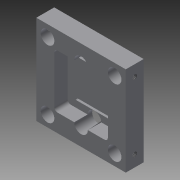
# Autodesk Inventor part: HolderEnd
Saved by Autodesk Inventor 2015 SP1 (Build 190203100, 203)
## iProperties
Created: 2014-07-11
Part Number: HolderEnd
Material: Generic
Document SubType Name: Modeling
Designer: jad211
Density: 1 g/cm^3
Appearance: Default
Author: jad211
Autodesk Inventor part; units mm, degrees
ref_plane "YZ Plane" through (0, 0, 0) normal (1, 0, 0) x (0, 1, 0)
ref_plane "XZ Plane" through (0, 0, 0) normal (0, 1, 0) x (-1, 0, 0)
ref_plane "XY Plane" through (0, 0, 0) normal (0, 0, 1) x (1, 0, 0)
sketch "Sketch1" plane through (0, 0, 0) normal (0, 1, 0) x (-1, 0, 0)
  line L0 (20, 20) -> (20, -20)
  line L1 (20, -20) -> (-20, -20)
  line L2 (-20, -20) -> (-20, 20)
  line L3 (-20, 20) -> (20, 20)
  line L4 (-15, 15) -> (-15, -15) construction
  line L5 (-15, -15) -> (15, -15) construction
  line L6 (15, -15) -> (15, 15) construction
  line L7 (15, 15) -> (-15, 15) construction
  circle A0 centre (15, 15) radius 3.05
  circle A1 centre (15, -15) radius 3.05
  circle A2 centre (-15, -15) radius 3.05
  circle A3 centre (-15, 15) radius 3.05
  line L8 (0, 0) -> (-18.5703, 0) construction
  line L9 (0, 0) -> (0, 18.05) construction
  line L10 (0, 0) -> (-18.05, 0) construction
  line L11 (8, 9) -> (-8, 9)
  line L12 (-8.5, 8.5) -> (-8.5, 8.5)
  line L13 (-8, 8) -> (8, 8)
  line L14 (8.5, 8.5) -> (8.5, 8.5)
  line L15 (8.5, 9) -> (-8.5, 8) construction
  line L16 (-8.5, 9) -> (8.5, 8) construction
  arc A4 (8.5, 8.5) -> (8, 9) centre (8, 8.5) ccw
  arc A5 (8, 8) -> (8.5, 8.5) centre (8, 8.5) ccw
  arc A6 (-8.5, 8.5) -> (-8, 8) centre (-8, 8.5) ccw
  arc A7 (-8, 9) -> (-8.5, 8.5) centre (-8, 8.5) ccw
  line L17 (8, -8) -> (-8, -8)
  line L18 (-8, -9) -> (8, -9)
  line L19 (8.5, -8) -> (-8.5, -9) construction
  line L20 (-8.5, -8) -> (8.5, -9) construction
  arc A8 (8.5, -8.5) -> (8, -8) centre (8, -8.5) ccw
  arc A9 (8, -9) -> (8.5, -8.5) centre (8, -8.5) ccw
  arc A10 (-8.5, -8.5) -> (-8, -9) centre (-8, -8.5) ccw
  arc A11 (-8, -8) -> (-8.5, -8.5) centre (-8, -8.5) ccw
  point P0 (0, -12.01)
  point P1 (0, 8.5)
  point P2 (0, 8.5)
  point P3 (0, -8.5)
  point P4 (0, -8.5)
  point P5 (0, -8.5)
  dimension "d118" = 17
  dimension "d0" = 40
  dimension "d1" = 40
  dimension "d2" = 30
  dimension "d53" = 20
  dimension "d114" = 17
  dimension "d115" = 1
  dimension "d116" = 8
  dimension "d117" = 0.5
  dimension "d119" = 1
  dimension "d120" = 0.5
  dimension "d121" = 16
  constraints: 42 end point, 16 point on circle, 15 point on line, 12 centre point, 12 tangent, 9 equal radius, 9 perpendicular, 7 horizontal, 7 midpoint, 4 coincident, 1 vertical, 14 other
  measures "d0" distance of L0.end L1.end
  measures "d1" distance of L0.start L0.end
  measures "d2" distance of L5.end L6.end
  measures "d53" distance from line of L8.start L1
  measures "d114" distance between parallel lines of L12 L14
  measures "d115" distance between parallel lines of L11 L13
  measures "d116" distance from line of L8.start L13
  measures "d117" radius of A4
  measures "d119" distance between parallel lines of L17 L18
  measures "d120" radius of A8
  measures "d121" distance between parallel lines of L13 L17
extrude "Extrusion11" add sketch "Sketch1" along normal blind 5
sketch "Sketch11" plane through (0, 0, 0) normal (0, -1, 0) x (1, 0, 0)
  line L0 (-10.5, -12) -> (10.5, -12)
  line L1 (12, -10.5) -> (12, 10.5)
  line L2 (10.5, 12) -> (-10.5, 12)
  line L3 (-12, 10.5) -> (-12, -10.5)
  line L4 (-12, -12) -> (12, 12) construction
  line L5 (12, -12) -> (-12, 12) construction
  arc A0 (-10.5, 12) -> (-12, 10.5) centre (-10.5, 10.5) ccw
  arc A1 (-12, -10.5) -> (-10.5, -12) centre (-10.5, -10.5) ccw
  arc A2 (10.5, -12) -> (12, -10.5) centre (10.5, -10.5) ccw
  arc A3 (12, 10.5) -> (10.5, 12) centre (10.5, 10.5) ccw
  point P0 (0, 0)
  dimension "d140" = 24
  dimension "d141" = 24
  dimension "d142" = 1.5
  constraints: 12 end point, 8 point on circle, 8 point on line, 8 tangent, 4 centre point, 3 equal radius, 2 midpoint, 2 perpendicular, 1 horizontal
  measures "d140" distance of L5.start L4.end
  measures "d141" distance of L4.end L5.end
  measures "d142" radius of A0
extrude "Extrusion14" cut sketch "Sketch11" against normal blind 3
sketch "Sketch14" plane through (0, 0, 0) normal (0, -1, 0) x (1, 0, 0)
  arc A0 (-12, -10.5) -> (-10.5, -12) centre (-10.5, -10.5) ccw projected
  line L0 (-12, -10.5) -> (-12, 10.5) projected
  arc A1 (-10.5, 12) -> (-12, 10.5) centre (-10.5, 10.5) ccw projected
  line L1 (-10.5, 12) -> (10.5, 12) projected
  arc A2 (12, 10.5) -> (10.5, 12) centre (10.5, 10.5) ccw projected
  line L2 (12, 10.5) -> (12, -10.5) projected
  arc A3 (10.5, -12) -> (12, -10.5) centre (10.5, -10.5) ccw projected
  line L3 (10.5, -12) -> (-10.5, -12) projected
  circle A4 centre (15, 15) radius 3.05 projected
  circle A5 centre (15, -15) radius 3.05 projected
  circle A6 centre (-15, -15) radius 3.05 projected
  circle A7 centre (-15, 15) radius 3.05 projected
  line L4 (-20, 20) -> (-20, -20) projected
  line L5 (-20, -20) -> (20, -20) projected
  line L6 (20, -20) -> (20, 20) projected
  line L7 (20, 20) -> (-20, 20) projected
  line L8 (8, 9) -> (-8, 9) projected
  line L9 (-8, -9) -> (8, -9) projected
  point P0 (0, 0)
extrude "Extrusion15" add sketch "Sketch14" along normal blind 3
sketch "Sketch12" plane through (20, 0, 20) normal (1, 0, 0) x (0, 0, -1)
  line L0 (40, 5) -> (40, -3) projected
  line L1 (0, 5) -> (40, 5) projected
  line L2 (0, 5) -> (0, -3) projected
  line L3 (40, -3) -> (0, -3) projected
  point P0 (20, 0)
  point P1 (5, 1)
  point P2 (35, 1)
  dimension "d145" = 5
  dimension "d148" = 5
  dimension "d167" = 4
  dimension "d168" = 4
  measures "d145" distance from line of L2 point (5, 1)
  measures "d148" distance from line of L0 point (35, 1)
  measures "d167" distance from line of L1 point (5, 1)
  measures "d168" distance from line of L1 point (35, 1)
hole "Hole1" at (20, 1, 15) at (20, 1, -15) direction (-1, 0, 0) diameter 2.013 depth 5 tip angle 118 thread size "M2.5x0.45" class "6H" standard "ISO Metric profile"
sketch "Sketch13" plane through (-20, 0, -20) normal (-1, 0, 0) x (0, 0, 1)
  line L0 (40, 0) -> (0, 0) projected
  line L1 (40, 0) -> (40, 5) projected
  circle A0 centre (5, 1) radius 1.0065 projected
  point P0 (20, 0)
  point P1 (35, 1)
  dimension "d156" = 1
  dimension "d157" = 5
  constraints: 1 coincident, 1 horizontal alignment, 2 other
  measures "d156" distance from line of L0 point (35, 1)
  measures "d157" distance from line of point (35, 1) L1
hole "Hole2" at (-20, 1, 15) at (-20, 1, -15) direction (1, 0, 0) diameter 2.013 depth 5 tip angle 118 thread size "M2.5x0.45" class "6H" standard "ISO Metric profile"
sketch "Sketch15" plane through (0, 5, 0) normal (0, 1, 0) x (1, 0, 0)
  circle A0 centre (0, -12.05) radius 3.05
  line L0 (8, -9) -> (-8, -9) projected
  circle A1 centre (0, 12.05) radius 3.05
  line L1 (-8, 9) -> (8, 9) projected
  point P0 (0, 0)
  dimension "d173" = 6.1
  dimension "d174" = 3.05
  dimension "d175" = 6.1
  dimension "d176" = 3.05
  constraints: 2 centre point
  measures "d173" diameter of A0
  measures "d174" distance from line of L0 A0.centre
  measures "d175" diameter of A1
  measures "d176" distance from line of L1 A1.centre
extrude "Extrusion16" cut sketch "Sketch15" against normal blind 10
equation "\"d1\" = d0"
body "Solid4"
